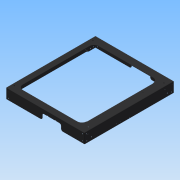
# Autodesk Inventor part: верхняя база
Saved by Autodesk Inventor 2017 (Build 210142000, 142)
## iProperties
Part Number: верхняя база
Material: Типовые
Document SubType Name: Modeling
Designer: Max
Mass: 130.784 g
Surface Area: 1912.46 cm^2
Volume: 130.784 cm^3
Density: 1 g/cm^3
Appearance: Резина — черная
Author: Max
Autodesk Inventor part; units mm, degrees
ref_plane "YZ Plane" through (0, 0, 0) normal (1, 0, 0) x (0, 1, 0)
ref_plane "XZ Plane" through (0, 0, 0) normal (0, 1, 0) x (-1, 0, 0)
ref_plane "XY Plane" through (0, 0, 0) normal (0, 0, 1) x (1, 0, 0)
sketch "Эскиз1" plane through (0, 0, 0) normal (0, 0, 1) x (1, 0, 0)
  line L0 (0, 0) -> (332.7, 0)
  line L1 (332.7, 0) -> (332.7, -378.7)
  line L2 (332.7, -378.7) -> (0, -378.7)
  line L3 (0, -378.7) -> (0, 0)
  line L4 (295.5, -31.2) -> (25, -31.2)
  line L5 (25, -31.2) -> (25, -352.7)
  line L6 (25, -352.7) -> (295.5, -352.7)
  line L7 (295.5, -352.7) -> (295.5, -31.2)
  line L8 (331.3, -1.4) -> (1.4, -1.4)
  line L9 (1.4, -1.4) -> (1.4, -377.3)
  line L10 (1.4, -377.3) -> (331.3, -377.3)
  line L11 (331.3, -377.3) -> (331.3, -1.4)
  dimension "d0" = 378.7
  dimension "d1" = 332.7
  dimension "d2" = 321.5
  dimension "d3" = 270.5
  dimension "d4" = 26
  dimension "d5" = 31.2
  dimension "d6" = 37.2
  dimension "d7" = 25
  dimension "d10" = 1.4
  constraints: 24 end point, 6 parallel, 3 perpendicular, 2 horizontal, 3 other
  measures "d0" distance between parallel lines of L2 L0
  measures "d1" distance between parallel lines of L3 L1
  measures "d2" distance between parallel lines of L4 L6
  measures "d3" distance between parallel lines of L5 L7
  measures "d4" distance between parallel lines of L2 L6
  measures "d5" distance between parallel lines of L0 L4
  measures "d6" distance between parallel lines of L7 L1
  measures "d7" distance between parallel lines of L3 L5
  measures "d10" distance between parallel lines of L0 L8
extrude "Выдавливание1" add sketch "Эскиз1" against normal blind 1.4 contours L0 L1 L2 L3 | L11 L10 L9 L8
extrude "Выдавливание2" add sketch "Эскиз1" against normal blind 42 contours L0 L1 L2 L3
fillet "Сопряжение1" radius 2 8 edges at (0, 0, -21) (166.35, 0, 0) (166.35, -378.7, 0) (0, -378.7, -21) (332.7, -378.7, -21) (332.7, -189.35, 0) (332.7, 0, -21) (0, -189.35, 0)
fillet "Сопряжение2" radius 0.6 8 edges at (1.4, -189.35, -1.4) (1.4, -1.4, -21.7) (166.35, -1.4, -1.4) (331.3, -1.4, -21.7) (331.3, -189.35, -1.4) (331.3, -377.3, -21.7) (1.4, -377.3, -21.7) (166.35, -377.3, -1.4)
sketch "Эскиз2" plane through (0, -376.7, -42) normal (-1, 0, 0) x (0, 0, 1)
  line L0 (0, 0) -> (0, 374.7) projected
  line L1 (0, 346.7) -> (4, 336.7)
  line L2 (4, 336.7) -> (4, 38)
  line L3 (4, 38) -> (0, 28)
  line L4 (0, 28) -> (0, 346.7)
  line L5 (40, 376.7) -> (0, 376.7) projected
  line L6 (0, -2) -> (40, -2) projected
  line L7 (42, 24) -> (42, 345.5) projected
  point P0 (42, 376.7)
  dimension "d15" = 30
  dimension "d16" = 40
  dimension "d17" = 30
  dimension "d18" = 40
  dimension "d19" = 38
  constraints: 8 end point, 2 parallel, 2 point on line
  measures "d15" distance from line of L1.start L5
  measures "d16" distance from line of L5 L1.end
  measures "d17" distance from line of L6 L3.end
  measures "d18" distance from line of L6 L2.end
  measures "d19" distance between parallel lines of L7 L2
extrude "Выдавливание3" cut sketch "Эскиз2" against normal blind 2
fillet "Сопряжение3" radius 10 4 edges at (0.7, -30, -42) (0.7, -40, -38) (0.7, -338.7, -38) (0.7, -348.7, -42)
sketch "Эскиз3" plane through (2, -378.7, -42) normal (0, -1, 0) x (1, 0, 0)
  line L0 (328.7, 0) -> (0, 0) projected
  line L1 (151.35, 0) -> (231.35, 0)
  line L2 (231.35, 0) -> (231.35, 24.5)
  line L3 (231.35, 24.5) -> (151.35, 24.5)
  line L4 (151.35, 24.5) -> (151.35, 0)
  line L5 (16.35, -307.35) -> (16.35, 42) projected
  line L6 (312.35, -307.35) -> (312.35, 42) projected
  circle A0 centre (174.35, 24.5) radius 2
  circle A1 centre (208.35, 24.5) radius 2
  point P0 (-2, 42)
  dimension "d23" = 135
  dimension "d24" = 81
  dimension "d25" = 24.5
  dimension "d26" = 80
  dimension "d30" = 4
  dimension "d31" = 4
  dimension "d32" = 34
  dimension "d33" = 23
  dimension "d34" = 23
  constraints: 8 end point, 3 point on line, 2 centre point, 2 parallel, 1 horizontal, 1 perpendicular
  measures "d23" distance between parallel lines of L5 L4
  measures "d24" distance between parallel lines of L6 L2
  measures "d25" distance between parallel lines of L0 L3
  measures "d26" distance between parallel lines of L2 L4
  measures "d30" diameter of A0
  measures "d31" diameter of A1
  measures "d32" distance of A1.centre A0.centre
  measures "d33" distance from line of L4 A0.centre
  measures "d34" distance of L2.end A1.centre
extrude "Выдавливание4" cut sketch "Эскиз3" against normal blind 500
fillet "Сопряжение4" radius 7 8 edges at (233.35, -378, -17.5) (233.35, -378, -42) (153.35, -378, -17.5) (153.35, -378, -42) (233.35, -0.7, -17.5) (233.35, -0.7, -42) (153.35, -0.7, -17.5) (153.35, -0.7, -42)
fillet "Сопряжение5" radius 20 4 edges at (25, -352.7, -0.7) (295.5, -352.7, -0.7) (295.5, -31.2, -0.7) (25, -31.2, -0.7)
sketch "Эскиз4" plane through (0, -376.7, -2) normal (-1, 0, 0) x (0, 0, 1)
  circle A0 centre (-6, 368.35) radius 2 projected
  circle A1 centre (-33, 366.35) radius 2 projected
  circle A2 centre (-6, 6.35) radius 2 projected
  circle A3 centre (-33, 8.35) radius 2 projected
  point P0 (2, 376.7)
extrude "Выдавливание5" cut sketch "Эскиз4" against normal blind 500
sketch "Эскиз5" plane through (2, -378.7, -2) normal (0, -1, 0) x (1, 0, 0)
  circle A0 centre (6.35, -6) radius 2 projected
  circle A1 centre (8.35, -33) radius 2 projected
  circle A2 centre (322.35, -6) radius 2 projected
  circle A3 centre (320.35, -33) radius 2 projected
  point P0 (-2, 2)
extrude "Выдавливание6" cut sketch "Эскиз5" against normal blind 500
sketch "Эскиз6" plane through (0, 0, -1.4) normal (0, 0, -1) x (-1, 0, 0)
  line L0 (-295.5, -332.7) -> (-295.5, -51.2) projected
  line L1 (-295.5, -51.2) -> (-296.9, -51.2)
  line L2 (-296.9, -51.2) -> (-296.9, -332.7)
  line L3 (-296.9, -332.7) -> (-295.5, -332.7)
  line L4 (-295.5, -332.7) -> (-295.5, -51.2)
  point P0 (0, 0)
  dimension "d40" = 1.4
  constraints: 8 end point, 2 parallel, 1 horizontal, 1 perpendicular
  measures "d40" distance between parallel lines of L0 L2
extrude "Выдавливание7" add sketch "Эскиз6" along normal blind 10.6
fillet "Сопряжение6" radius 4 2 edges at (296.2, -51.2, -12) (296.2, -332.7, -12)
sketch "Эскиз7" plane through (0, 0, 0) normal (0, 0, 1) x (1, 0, 0)
  line L0 (295.5, -55.2) -> (295.5, -51.2) projected
  line L1 (295.5, -51.2) -> (297.5, -51.2)
  line L2 (297.5, -51.2) -> (297.5, -51)
  line L3 (297.5, -51) -> (295.5, -51)
  line L4 (295.5, -51) -> (295.5, -51.2)
  line L5 (295.5, -51) -> (295.356, -51)
  line L6 (295.356, -51) -> (295.356, -51.2)
  line L7 (295.356, -51.2) -> (295.5, -51.2)
  line L8 (295.5, -51.2) -> (295.5, -51)
  line L9 (295.5, -332.7) -> (296.9, -332.7) projected
  line L10 (295.5, -332.7) -> (297.5, -332.7)
  line L11 (297.5, -332.7) -> (297.5, -332.9)
  line L12 (297.5, -332.9) -> (291.4104, -332.9)
  line L13 (291.4104, -332.9) -> (291.4104, -332.7)
  line L14 (291.4104, -332.7) -> (295.5, -332.7)
  line L15 (295.5, -51.2) -> (295.5, -332.7) projected
  point P0 (0, 0)
  dimension "d44" = 2
  dimension "d45" = 0.2
  dimension "d46" = 2
  dimension "d47" = 0.2
  constraints: 26 end point, 5 perpendicular, 4 parallel, 3 horizontal, 1 collinear
  measures "d44" distance of L3.end L2.end
  measures "d45" distance between parallel lines of L12 L9
  measures "d46" distance from line of L10.end L15
  measures "d47" distance between parallel lines of L1 L3
extrude "Выдавливание8" cut sketch "Эскиз7" against normal blind 10.6
fillet "Сопряжение7" radius 2 1 edges at (295.5, -191.95, 0)
sketch "Эскиз8" plane through (0, -376.7, -2) normal (-1, 0, 0) x (0, 0, 1)
  circle A0 centre (-10.5, 338.9) radius 1.5
  line L0 (2, 0) -> (2, 374.7) projected
  circle A1 centre (-10.5, 338.9) radius 4 construction
  line L1 (0, 376.7) -> (-40, 376.7) projected
  circle A2 centre (-10.5, 12.9) radius 1.5
  circle A3 centre (-10.5, 12.9) radius 4 construction
  point P0 (2, 376.7)
  dimension "d51" = 3
  dimension "d52" = 12.5
  dimension "d53" = 8
  dimension "d54" = 41.8
  dimension "d55" = 3
  dimension "d56" = 8
  dimension "d57" = 12.5
  dimension "d58" = 326
  dimension "d59" = 318
  constraints: 4 centre point, 2 coincident
  measures "d51" diameter of A0
  measures "d52" distance from line of A0.centre L0
  measures "d53" diameter of A1
  measures "d55" diameter of A2
  measures "d56" diameter of A3
  measures "d57" distance from line of L0 A2.centre
  measures "d58" distance of A0.centre A2.centre
extrude "Выдавливание9" cut sketch "Эскиз8" against normal blind 600
sketch "Эскиз9" plane through (0, -376.7, -2) normal (-1, 0, 0) x (0, 0, 1)
  line L0 (-11.5044, 298.2897) -> (-11.5044, -254.3895) construction
  line L1 (-11.5044, -254.3895) -> (-54.8278, -254.3895) construction
  line L2 (-54.8278, -254.3895) -> (-54.8278, 298.2897) construction
  line L3 (-54.8278, 298.2897) -> (-11.5044, 298.2897) construction
  line L4 (-11.7296, 296.9384) -> (-11.7296, 287.0164)
  line L5 (-11.7296, 287.0164) -> (-14.5198, 287.0164)
  line L6 (-14.5198, 287.0164) -> (-14.5198, 292.8971)
  line L7 (-14.5198, 292.8971) -> (-16.7844, 292.8971)
  line L8 (-16.7844, 292.8971) -> (-16.7844, 287.8797)
  line L9 (-16.7844, 287.8797) -> (-19.412, 287.8797)
  line L10 (-19.412, 287.8797) -> (-19.412, 292.8971)
  line L11 (-19.412, 292.8971) -> (-24.7296, 292.8971)
  line L12 (-24.7296, 292.8971) -> (-24.7296, 296.9384)
  line L13 (-24.7296, 296.9384) -> (-11.7296, 296.9384)
  line L14 (-11.7296, 284.8393) -> (-11.7296, 280.8229)
  line L15 (-11.7296, 280.8229) -> (-21.5265, 280.8229)
  line L16 (-21.5265, 280.8229) -> (-21.5265, 274.5544)
  line L17 (-21.5265, 274.5544) -> (-24.7296, 274.5544)
  line L18 (-24.7296, 274.5544) -> (-24.7296, 284.8393)
  line L19 (-24.7296, 284.8393) -> (-11.7296, 284.8393)
  line L20 (-11.7296, 274.0289) -> (-11.7296, 269.5621)
  line L21 (-11.7296, 269.5621) -> (-16.1088, 266.9471)
  line L22 (-16.1088, 266.9471) -> (-11.7296, 264.3196)
  line L23 (-11.7296, 264.3196) -> (-11.7296, 259.8778)
  line L24 (-11.7296, 259.8778) -> (-19.2869, 264.9327)
  line L25 (-19.2869, 264.9327) -> (-24.7296, 264.9327)
  line L26 (-24.7296, 264.9327) -> (-24.7296, 268.9615)
  line L27 (-24.7296, 268.9615) -> (-19.2869, 268.9615)
  line L28 (-19.2869, 268.9615) -> (-11.7296, 274.0289)
  line L29 (-11.7296, 258.4139) -> (-11.7296, 254.385)
  line L30 (-11.7296, 254.385) -> (-24.7296, 254.385)
  line L31 (-24.7296, 254.385) -> (-24.7296, 258.4139)
  line L32 (-24.7296, 258.4139) -> (-11.7296, 258.4139)
  line L33 (-11.7296, 251.4822) -> (-11.7296, 247.7286)
  line L34 (-11.7296, 247.7286) -> (-18.924, 242.8239)
  line L35 (-18.924, 242.8239) -> (-11.7296, 242.8239)
  line L36 (-11.7296, 242.8239) -> (-11.7296, 239.0328)
  line L37 (-11.7296, 239.0328) -> (-24.7296, 239.0328)
  line L38 (-24.7296, 239.0328) -> (-24.7296, 242.8239)
  line L39 (-24.7296, 242.8239) -> (-17.5727, 247.7036)
  line L40 (-17.5727, 247.7036) -> (-24.7296, 247.7036)
  line L41 (-24.7296, 247.7036) -> (-24.7296, 251.4822)
  line L42 (-24.7296, 251.4822) -> (-11.7296, 251.4822)
  line L43 (-20.0251, 229.8114) -> (-17.3225, 229.8114)
  line L44 (-17.3225, 229.8114) -> (-17.3225, 223.6054)
  line L45 (-17.3225, 223.6054) -> (-22.8528, 223.6054)
  spline S0 degree 2 poles (-22.8528, 223.6054) (-24.079, 225.3946) (-24.9548, 228.1348) (-24.9548, 230.0116) knots 0 0 0 1 2 2 2
  spline S1 degree 2 poles (-24.9548, 230.0116) (-24.9548, 232.3263) (-23.3783, 235.2541) (-20.2503, 236.8557) (-18.2233, 236.8557) knots 0 0 0 1 2 3 3 3
  spline S2 degree 2 poles (-18.2233, 236.8557) (-16.0963, 236.8557) (-12.9558, 235.104) (-12.13, 233.4023) knots 0 0 0 1 2 2 2
  spline S3 degree 2 poles (-12.13, 233.4023) (-11.5044, 232.0761) (-11.5044, 229.8489) knots 0 0 0 1 1 1
  spline S4 degree 2 poles (-11.5044, 229.8489) (-11.5044, 227.6844) (-12.2801, 225.5448) (-13.9317, 224.1309) (-15.1829, 223.7806) knots 0 0 0 1 2 3 3 3
  line L46 (-15.1829, 223.7806) -> (-15.8836, 227.6593)
  spline S5 degree 2 poles (-15.8836, 227.6593) (-15.1454, 227.8971) (-14.3571, 229.0482) (-14.3571, 229.9365) knots 0 0 0 1 2 2 2
  spline S6 degree 2 poles (-14.3571, 229.9365) (-14.3571, 231.2503) (-16.1964, 232.8268) (-18.1858, 232.8268) knots 0 0 0 1 2 2 2
  spline S7 degree 2 poles (-18.1858, 232.8268) (-20.2878, 232.8268) (-22.1021, 231.2378) (-22.1021, 229.8114) knots 0 0 0 1 2 2 2
  spline S8 degree 2 poles (-22.1021, 229.8114) (-22.1021, 229.1357) (-21.7142, 227.9096) (-21.2387, 227.1213) knots 0 0 0 1 2 2 2
  line L47 (-21.2387, 227.1213) -> (-20.0251, 227.1213)
  line L48 (-20.0251, 227.1213) -> (-20.0251, 229.8114)
  line L49 (-11.7296, 215.1598) -> (-11.7296, 207.6401)
  spline S9 degree 2 poles (-11.7296, 207.6401) (-11.7296, 205.7633) (-13.5939, 203.7488) (-14.9702, 203.7488) knots 0 0 0 1 2 2 2
  spline S10 degree 2 poles (-14.9702, 203.7488) (-16.1213, 203.7488) (-16.9471, 204.462) knots 0 0 0 1 1 1
  spline S11 degree 2 poles (-16.9471, 204.462) (-17.4976, 204.95) (-17.8229, 205.8759) knots 0 0 0 1 1 1
  spline S12 degree 2 poles (-17.8229, 205.8759) (-18.1608, 204.4745) (-19.7998, 203.1483) (-21.0385, 203.1483) knots 0 0 0 1 2 2 2
  spline S13 degree 2 poles (-21.0385, 203.1483) (-22.0395, 203.1483) (-23.6536, 204.0867) (-24.129, 204.8999) knots 0 0 0 1 2 2 2
  spline S14 degree 2 poles (-24.129, 204.8999) (-24.4168, 205.4129) (-24.5544, 206.4264) knots 0 0 0 1 1 1
  spline S15 degree 2 poles (-24.5544, 206.4264) (-24.7296, 207.7902) (-24.7296, 208.2281) knots 0 0 0 1 1 1
  line L50 (-24.7296, 208.2281) -> (-24.7296, 215.1598)
  line L51 (-24.7296, 215.1598) -> (-11.7296, 215.1598)
  line L52 (-21.9394, 211.1059) -> (-21.9394, 209.0664)
  spline S16 degree 2 poles (-21.9394, 209.0664) (-21.9394, 208.028) (-21.2012, 207.1771) (-20.5881, 207.1771) knots 0 0 0 1 2 2 2
  spline S17 degree 2 poles (-20.5881, 207.1771) (-20.0126, 207.1771) (-19.3119, 208.0154) (-19.3119, 209.0664) knots 0 0 0 1 2 2 2
  line L53 (-19.3119, 209.0664) -> (-19.3119, 211.1059)
  line L54 (-19.3119, 211.1059) -> (-21.9394, 211.1059)
  line L55 (-16.8345, 211.1059) -> (-16.8345, 209.3667)
  spline S18 degree 2 poles (-16.8345, 209.3667) (-16.8345, 208.4283) (-16.1839, 207.6901) (-15.5708, 207.6901) knots 0 0 0 1 2 2 2
  spline S19 degree 2 poles (-15.5708, 207.6901) (-15.0077, 207.6901) (-14.3696, 208.4283) (-14.3696, 209.3417) knots 0 0 0 1 2 2 2
  line L56 (-14.3696, 209.3417) -> (-14.3696, 211.1059)
  line L57 (-14.3696, 211.1059) -> (-16.8345, 211.1059)
  line L58 (-11.7296, 201.0337) -> (-11.7296, 190.2734)
  line L59 (-11.7296, 190.2734) -> (-14.5073, 190.2734)
  line L60 (-14.5073, 190.2734) -> (-14.5073, 197.0049)
  line L61 (-14.5073, 197.0049) -> (-16.5717, 197.0049)
  line L62 (-16.5717, 197.0049) -> (-16.5717, 190.7613)
  line L63 (-16.5717, 190.7613) -> (-19.2243, 190.7613)
  line L64 (-19.2243, 190.7613) -> (-19.2243, 197.0049)
  line L65 (-19.2243, 197.0049) -> (-21.7893, 197.0049)
  line L66 (-21.7893, 197.0049) -> (-21.7893, 190.0732)
  line L67 (-21.7893, 190.0732) -> (-24.7296, 190.0732)
  line L68 (-24.7296, 190.0732) -> (-24.7296, 201.0337)
  line L69 (-24.7296, 201.0337) -> (-11.7296, 201.0337)
  line L70 (-22.5775, 179.9134) -> (-22.5775, 184.4803)
  line L71 (-22.5775, 184.4803) -> (-24.7296, 185.1184)
  line L72 (-24.7296, 185.1184) -> (-24.7296, 189.2224)
  line L73 (-24.7296, 189.2224) -> (-11.7296, 184.3302)
  line L74 (-11.7296, 184.3302) -> (-11.7296, 179.9384)
  line L75 (-11.7296, 179.9384) -> (-24.7296, 175.0588)
  line L76 (-24.7296, 175.0588) -> (-24.7296, 179.2628)
  line L77 (-24.7296, 179.2628) -> (-22.5775, 179.9134)
  line L78 (-19.7623, 180.7517) -> (-15.0953, 182.1781)
  line L79 (-15.0953, 182.1781) -> (-19.7623, 183.6045)
  line L80 (-19.7623, 183.6045) -> (-19.7623, 180.7517)
  line L81 (-24.7296, 173.7075) -> (-11.7296, 173.7075)
  line L82 (-11.7296, 173.7075) -> (-11.7296, 167.0135)
  spline S20 degree 2 poles (-11.7296, 167.0135) (-11.7296, 165.1617) (-12.3677, 163.1848) (-14.0944, 161.9837) (-15.3331, 161.9837) knots 0 0 0 1 2 3 3 3
  spline S21 degree 2 poles (-15.3331, 161.9837) (-16.4216, 161.9837) (-17.9856, 162.9096) (-18.4736, 163.7103) knots 0 0 0 1 2 2 2
  spline S22 degree 2 poles (-18.4736, 163.7103) (-18.7864, 164.2233) (-18.9866, 165.1242) knots 0 0 0 1 1 1
  spline S23 degree 2 poles (-18.9866, 165.1242) (-19.2243, 164.411) (-19.462, 164.0732) knots 0 0 0 1 1 1
  spline S24 degree 2 poles (-19.462, 164.0732) (-19.6247, 163.8605) (-20.6757, 163.0222) (-20.9635, 162.872) knots 0 0 0 1 2 2 2
  line L83 (-20.9635, 162.872) -> (-24.7296, 160.9327)
  line L84 (-24.7296, 160.9327) -> (-24.7296, 165.4745)
  line L85 (-24.7296, 165.4745) -> (-20.7508, 167.6141)
  spline S25 degree 2 poles (-20.7508, 167.6141) (-19.9875, 168.0145) (-19.7498, 168.3273) knots 0 0 0 1 1 1
  spline S26 degree 2 poles (-19.7498, 168.3273) (-19.4495, 168.7652) (-19.4495, 169.3157) knots 0 0 0 1 1 1
  line L86 (-19.4495, 169.3157) -> (-19.4495, 169.6661)
  line L87 (-19.4495, 169.6661) -> (-24.7296, 169.6661)
  line L88 (-24.7296, 169.6661) -> (-24.7296, 173.7075)
  line L89 (-16.9972, 169.6661) -> (-16.9972, 167.9769)
  spline S27 degree 2 poles (-16.9972, 167.9769) (-16.9972, 167.7142) (-16.822, 166.9259) knots 0 0 0 1 1 1
  spline S28 degree 2 poles (-16.822, 166.9259) (-16.7344, 166.5255) (-16.0838, 166.0251) (-15.6584, 166.0251) knots 0 0 0 1 2 2 2
  spline S29 degree 2 poles (-15.6584, 166.0251) (-15.0328, 166.0251) (-14.3571, 166.8133) (-14.3571, 167.9144) knots 0 0 0 1 2 2 2
  line L90 (-14.3571, 167.9144) -> (-14.3571, 169.6661)
  line L91 (-14.3571, 169.6661) -> (-16.9972, 169.6661)
  line L92 (-20.0251, 147.0193) -> (-17.3225, 147.0193)
  line L93 (-17.3225, 147.0193) -> (-17.3225, 140.8133)
  line L94 (-17.3225, 140.8133) -> (-22.8528, 140.8133)
  spline S30 degree 2 poles (-22.8528, 140.8133) (-24.079, 142.6025) (-24.9548, 145.3427) (-24.9548, 147.2195) knots 0 0 0 1 2 2 2
  spline S31 degree 2 poles (-24.9548, 147.2195) (-24.9548, 149.5342) (-23.3783, 152.462) (-20.2503, 154.0636) (-18.2233, 154.0636) knots 0 0 0 1 2 3 3 3
  spline S32 degree 2 poles (-18.2233, 154.0636) (-16.0963, 154.0636) (-12.9558, 152.3119) (-12.13, 150.6102) knots 0 0 0 1 2 2 2
  spline S33 degree 2 poles (-12.13, 150.6102) (-11.5044, 149.284) (-11.5044, 147.0568) knots 0 0 0 1 1 1
  spline S34 degree 2 poles (-11.5044, 147.0568) (-11.5044, 144.8922) (-12.2801, 142.7527) (-13.9317, 141.3388) (-15.1829, 140.9885) knots 0 0 0 1 2 3 3 3
  line L95 (-15.1829, 140.9885) -> (-15.8836, 144.8672)
  spline S35 degree 2 poles (-15.8836, 144.8672) (-15.1454, 145.105) (-14.3571, 146.2561) (-14.3571, 147.1444) knots 0 0 0 1 2 2 2
  spline S36 degree 2 poles (-14.3571, 147.1444) (-14.3571, 148.4582) (-16.1964, 150.0347) (-18.1858, 150.0347) knots 0 0 0 1 2 2 2
  spline S37 degree 2 poles (-18.1858, 150.0347) (-20.2878, 150.0347) (-22.1021, 148.4457) (-22.1021, 147.0193) knots 0 0 0 1 2 2 2
  spline S38 degree 2 poles (-22.1021, 147.0193) (-22.1021, 146.3436) (-21.7142, 145.1175) (-21.2387, 144.3292) knots 0 0 0 1 2 2 2
  line L96 (-21.2387, 144.3292) -> (-20.0251, 144.3292)
  line L97 (-20.0251, 144.3292) -> (-20.0251, 147.0193)
  line L98 (-11.7296, 138.411) -> (-11.7296, 134.3947)
  line L99 (-11.7296, 134.3947) -> (-16.284, 134.3947)
  line L100 (-16.284, 134.3947) -> (-16.284, 130.0029)
  line L101 (-16.284, 130.0029) -> (-11.7296, 130.0029)
  line L102 (-11.7296, 130.0029) -> (-11.7296, 125.9615)
  line L103 (-11.7296, 125.9615) -> (-24.7296, 125.9615)
  line L104 (-24.7296, 125.9615) -> (-24.7296, 130.0029)
  line L105 (-24.7296, 130.0029) -> (-19.4745, 130.0029)
  line L106 (-19.4745, 130.0029) -> (-19.4745, 134.3947)
  line L107 (-19.4745, 134.3947) -> (-24.7296, 134.3947)
  line L108 (-24.7296, 134.3947) -> (-24.7296, 138.411)
  line L109 (-24.7296, 138.411) -> (-11.7296, 138.411)
  spline S39 degree 2 poles (-18.2358, 123.797) (-15.0578, 123.797) (-11.5044, 120.2435) (-11.5044, 117.078) knots 0 0 0 1 2 2 2
  spline S40 degree 2 poles (-11.5044, 117.078) (-11.5044, 113.8374) (-14.9952, 110.3215) (-18.1357, 110.3215) knots 0 0 0 1 2 2 2
  spline S41 degree 2 poles (-18.1357, 110.3215) (-20.4129, 110.3215) (-23.3282, 111.8605) (-24.9548, 114.7633) (-24.9548, 116.9279) knots 0 0 0 1 2 3 3 3
  spline S42 degree 2 poles (-24.9548, 116.9279) (-24.9548, 119.1175) (-23.5535, 122.0077) (-20.513, 123.797) (-18.2358, 123.797) knots 0 0 0 1 2 3 3 3
  spline S43 degree 2 poles (-18.2609, 119.7806) (-20.2253, 119.7806) (-21.9519, 118.3167) (-21.9519, 117.053) knots 0 0 0 1 2 2 2
  spline S44 degree 2 poles (-21.9519, 117.053) (-21.9519, 115.7642) (-20.2628, 114.3379) (-18.0857, 114.3379) knots 0 0 0 1 2 2 2
  spline S45 degree 2 poles (-18.0857, 114.3379) (-16.2464, 114.3379) (-14.5448, 115.8143) (-14.5448, 117.0905) knots 0 0 0 1 2 2 2
  spline S46 degree 2 poles (-14.5448, 117.0905) (-14.5448, 118.3042) (-16.2715, 119.7806) (-18.2609, 119.7806) knots 0 0 0 1 2 2 2
  line L110 (-20.4254, 108.8576) -> (-20.1877, 105.0289)
  spline S47 degree 2 poles (-20.1877, 105.0289) (-21.1261, 104.9038) (-21.6141, 104.5284) knots 0 0 0 1 1 1
  spline S48 degree 2 poles (-21.6141, 104.5284) (-22.4023, 103.9028) (-22.4023, 102.7392) knots 0 0 0 1 1 1
  spline S49 degree 2 poles (-22.4023, 102.7392) (-22.4023, 101.8884) (-21.5891, 100.95) (-21.0636, 100.95) knots 0 0 0 1 2 2 2
  spline S50 degree 2 poles (-21.0636, 100.95) (-20.5631, 100.95) (-20.1627, 101.4004) knots 0 0 0 1 1 1
  spline S51 degree 2 poles (-20.1627, 101.4004) (-19.7623, 101.8383) (-19.3995, 103.4524) knots 0 0 0 1 1 1
  spline S52 degree 2 poles (-19.3995, 103.4524) (-18.8114, 106.105) (-17.8229, 107.231) knots 0 0 0 1 1 1
  spline S53 degree 2 poles (-17.8229, 107.231) (-16.8345, 108.3696) (-15.308, 108.3696) knots 0 0 0 1 1 1
  spline S54 degree 2 poles (-15.308, 108.3696) (-14.3071, 108.3696) (-12.5304, 107.206) (-11.5044, 104.8663) (-11.5044, 102.8393) knots 0 0 0 1 2 3 3 3
  spline S55 degree 2 poles (-11.5044, 102.8393) (-11.5044, 100.3369) (-13.3562, 97.7219) (-15.3831, 97.4717) knots 0 0 0 1 2 2 2
  line L111 (-15.3831, 97.4717) -> (-15.6083, 101.2628)
  spline S56 degree 2 poles (-15.6083, 101.2628) (-14.7325, 101.4129) (-13.9317, 102.3889) (-13.9317, 103.2397) knots 0 0 0 1 2 2 2
  spline S57 degree 2 poles (-13.9317, 103.2397) (-13.9317, 103.9404) (-14.5198, 104.6536) (-14.9577, 104.6536) knots 0 0 0 1 2 2 2
  spline S58 degree 2 poles (-14.9577, 104.6536) (-15.258, 104.6536) (-15.5082, 104.3533) knots 0 0 0 1 1 1
  spline S59 degree 2 poles (-15.5082, 104.3533) (-15.771, 104.0655) (-15.9837, 103.002) knots 0 0 0 1 1 1
  spline S60 degree 2 poles (-15.9837, 103.002) (-16.5592, 100.3619) (-17.7229, 98.0847) (-19.437, 97.0462) (-20.5005, 97.0462) knots 0 0 0 1 2 3 3 3
  spline S61 degree 2 poles (-20.5005, 97.0462) (-21.7517, 97.0462) (-23.8663, 98.4351) (-24.9548, 100.9125) (-24.9548, 102.8143) knots 0 0 0 1 2 3 3 3
  spline S62 degree 2 poles (-24.9548, 102.8143) (-24.9548, 106.13) (-22.4023, 108.6949) (-20.4254, 108.8576) knots 0 0 0 1 2 2 2
  line L112 (-11.7296, 95.9452) -> (-11.7296, 83.7209)
  line L113 (-11.7296, 83.7209) -> (-14.9452, 83.7209)
  line L114 (-14.9452, 83.7209) -> (-14.9452, 87.8249)
  line L115 (-14.9452, 87.8249) -> (-24.7296, 87.8249)
  line L116 (-24.7296, 87.8249) -> (-24.7296, 91.8412)
  line L117 (-24.7296, 91.8412) -> (-14.9452, 91.8412)
  line L118 (-14.9452, 91.8412) -> (-14.9452, 95.9452)
  line L119 (-14.9452, 95.9452) -> (-11.7296, 95.9452)
  line L120 (-11.7296, 74.9625) -> (-11.7296, 66.4043)
  line L121 (-11.7296, 66.4043) -> (-14.6074, 66.4043)
  line L122 (-14.6074, 66.4043) -> (-14.6074, 72.1973)
  line L123 (-14.6074, 72.1973) -> (-16.5592, 72.4976)
  spline S63 degree 2 poles (-16.5592, 72.4976) (-16.284, 71.8971) (-15.9962, 70.7209) (-15.9962, 70.1454) knots 0 0 0 1 2 2 2
  spline S64 degree 2 poles (-15.9962, 70.1454) (-15.9962, 68.206) (-18.361, 65.7787) (-20.1502, 65.7787) knots 0 0 0 1 2 2 2
  spline S65 degree 2 poles (-20.1502, 65.7787) (-21.4014, 65.7787) (-23.7286, 67.0299) (-24.9548, 69.3196) (-24.9548, 71.1088) knots 0 0 0 1 2 3 3 3
  spline S66 degree 2 poles (-24.9548, 71.1088) (-24.9548, 72.3975) (-24.4668, 74.2243) (-23.5034, 75.513) (-22.2772, 76.3138) (-21.3639, 76.5766) knots 0 0 0 1 2 3 4 4 4
  line L124 (-21.3639, 76.5766) -> (-20.9635, 72.923)
  spline S67 degree 2 poles (-20.9635, 72.923) (-21.8393, 72.7854) (-22.7527, 71.822) (-22.7527, 71.1463) knots 0 0 0 1 2 2 2
  spline S68 degree 2 poles (-22.7527, 71.1463) (-22.7527, 70.3956) (-21.6141, 69.4197) (-20.4755, 69.4197) knots 0 0 0 1 2 2 2
  spline S69 degree 2 poles (-20.4755, 69.4197) (-19.3119, 69.4197) (-18.2358, 70.4081) (-18.2358, 71.2214) knots 0 0 0 1 2 2 2
  spline S70 degree 2 poles (-18.2358, 71.2214) (-18.2358, 71.7469) (-18.4986, 72.2349) knots 0 0 0 1 1 1
  spline S71 degree 2 poles (-18.4986, 72.2349) (-18.6738, 72.5852) (-19.1617, 73.0231) knots 0 0 0 1 1 1
  line L125 (-19.1617, 73.0231) -> (-18.7238, 76.1011)
  line L126 (-18.7238, 76.1011) -> (-11.7296, 74.9625)
  point P0 (2, 376.7)
  constraints: 2 other
extrude "Выдавливание10" add sketch "Эскиз9" along normal blind 0.1
sketch "Эскиз10" plane through (0, 0, 0) normal (0, 0, 1) x (1, 0, 0)
  circle A0 centre (308.35, -96.85) radius 6 projected
  circle A1 centre (308.35, -107.85) radius 1.5 projected
  circle A2 centre (308.35, -85.85) radius 1.5 projected
  circle A3 centre (308.35, -270.85) radius 1.5 projected
  circle A4 centre (308.35, -281.85) radius 6 projected
  circle A5 centre (308.35, -292.85) radius 1.5 projected
  line L0 (315.25, -295.85) -> (301.45, -295.85) projected
  line L1 (315.25, -110.85) -> (301.45, -110.85) projected
  line L2 (300.95, -110.35) -> (300.95, -83.35) projected
  line L3 (300.95, -295.35) -> (300.95, -268.35) projected
  line L4 (315.75, -268.35) -> (315.75, -295.35) projected
  line L5 (301.45, -267.85) -> (315.25, -267.85) projected
  line L6 (315.75, -83.35) -> (315.75, -110.35) projected
  line L7 (301.45, -82.85) -> (315.25, -82.85) projected
  point P0 (0, 0)
extrude "Выдавливание11" cut sketch "Эскиз10" against normal blind 5 contours A1 | A2 | A3 | A5
sketch "Эскиз11" plane through (0, -376.7, -2) normal (-1, 0, 0) x (0, 0, 1)
  circle A0 centre (-33.5, 354.7) radius 2
  circle A1 centre (-33.5, 21.7) radius 2
  line L0 (0, 376.7) -> (-40, 376.7) projected
  line L1 (-40, -2) -> (0, -2) projected
  line L2 (-47.7633, 16.35) -> (-56.1519, 16.35)
  line L3 (2, 0) -> (2, 374.7) projected
  point P0 (2, 376.7)
  dimension "d66" = 4
  dimension "d67" = 4
  dimension "d68" = 22
  dimension "d70" = 333
  dimension "d71" = 5.35
  dimension "d73" = 18.35
  dimension "d74" = 35.5
  dimension "d75" = 35.5
  dimension "d78" = 23.7
  constraints: 2 centre point, 2 end point, 1 horizontal
  measures "d66" diameter of A0
  measures "d67" diameter of A1
  measures "d68" distance from line of L0 A0.centre
  measures "d70" distance of A0.centre A1.centre
  measures "d71" distance from line of L2 A1.centre
  measures "d73" distance between parallel lines of L1 L2
  measures "d74" distance from line of A0.centre L3
  measures "d75" distance from line of L3 A1.centre
  measures "d78" distance from line of A1.centre L1
extrude "Выдавливание12" cut sketch "Эскиз11" against normal blind 5
sketch "Эскиз12" plane through (0, 0, 0) normal (0, 0, 1) x (1, 0, 0)
  circle A0 centre (11.5, -22) radius 2
  circle A1 centre (11.5, -355) radius 2
  line L0 (330.7, 0) -> (2, 0) projected
  line L1 (2, -378.7) -> (330.7, -378.7) projected
  line L2 (0, -2) -> (0, -376.7) projected
  circle A2 centre (318.2, -28) radius 2
  circle A3 centre (318.2, -348.7) radius 2
  line L3 (332.7, -376.7) -> (332.7, -2) projected
  point P0 (0, 0)
  dimension "d79" = 4
  dimension "d80" = 4
  dimension "d81" = 22
  dimension "d82" = 23.7
  dimension "d83" = 333
  dimension "d84" = 11.5
  dimension "d85" = 11.5
  dimension "d86" = 4
  dimension "d87" = 4
  dimension "d88" = 14.5
  dimension "d89" = 14.5
  dimension "d90" = 28
  dimension "d91" = 30
  constraints: 4 centre point
  measures "d79" diameter of A0
  measures "d80" diameter of A1
  measures "d81" distance from line of L0 A0.centre
  measures "d82" distance from line of L1 A1.centre
  measures "d83" distance of A0.centre A1.centre
  measures "d84" distance from line of L2 A0.centre
  measures "d85" distance from line of L2 A1.centre
  measures "d86" diameter of A2
  measures "d87" diameter of A3
  measures "d88" distance from line of L3 A3.centre
  measures "d89" distance from line of L3 A2.centre
  measures "d90" distance from line of L0 A2.centre
  measures "d91" distance from line of L1 A3.centre
extrude "Выдавливание13" cut sketch "Эскиз12" against normal blind 5
sketch "Эскиз13" plane through (332.7, -376.7, -2) normal (1, 0, 0) x (0, 0, -1)
  circle A0 centre (28, 348.7) radius 2
  line L0 (40, 376.7) -> (0, 376.7) projected
  line L1 (-2, 374.7) -> (-2, 0) projected
  circle A1 centre (28, 28) radius 2
  line L2 (0, -2) -> (40, -2) projected
  point P0 (-2, 376.7)
  dimension "d94" = 4
  dimension "d95" = 28
  dimension "d96" = 30
  dimension "d97" = 4
  dimension "d98" = 30
  dimension "d99" = 30
  constraints: 2 centre point
  measures "d94" diameter of A0
  measures "d95" distance from line of L0 A0.centre
  measures "d96" distance from line of L1 A0.centre
  measures "d97" diameter of A1
  measures "d98" distance from line of L2 A1.centre
  measures "d99" distance from line of A1.centre L1
extrude "Выдавливание14" cut sketch "Эскиз13" against normal blind 5
sketch "Эскиз14" plane through (1.4, -376.7, -2) normal (1, 0, 0) x (0, 0, -1)
  circle A0 centre (25.0596, 330.9914) radius 1.5 projected
  circle A1 centre (25.0596, 330.9914) radius 1
  point P0 (-2, 376.7)
  dimension "d104" = 2
  constraints: 1 centre point, 1 coincident
  measures "d104" diameter of A1
extrude "Выдавливание15" add sketch "Эскиз14" along normal blind 12
sketch "Эскиз15" plane through (332.7, -376.7, -2) normal (1, 0, 0) x (0, 0, -1)
  circle A0 centre (34, 135) radius 1.5
  circle A1 centre (34, 150) radius 1.5
  line L0 (-2, 374.7) -> (-2, 0) projected
  line L1 (0, -2) -> (40, -2) projected
  point P0 (-2, 376.7)
  dimension "d105" = 3
  dimension "d106" = 3
  dimension "d107" = 36
  dimension "d108" = 36
  dimension "d109" = 15
  dimension "d110" = 137
  constraints: 2 centre point
  measures "d105" diameter of A0
  measures "d106" diameter of A1
  measures "d107" distance from line of A1.centre L0
  measures "d108" distance from line of L0 A0.centre
  measures "d109" distance of A1.centre A0.centre
  measures "d110" distance from line of L1 A0.centre
extrude "Выдавливание16" cut sketch "Эскиз15" against normal blind 12
sketch "Эскиз16" plane through (332.7, -376.7, -2) normal (1, 0, 0) x (0, 0, -1)
  circle A0 centre (37, 187.85) radius 1.5
  line L0 (-2, 374.7) -> (-2, 0) projected
  circle A1 centre (45, 366.85) radius 1.1293 projected
  circle A2 centre (10.5, 338.9) radius 1.5 projected
  circle A3 centre (34, 150) radius 1.5 projected
  point P0 (-2, 376.7)
  dimension "d113" = 3
  dimension "d114" = 39
  dimension "d115" = 179
  dimension "d116" = 151.05
  dimension "d119" = 36
  constraints: 1 centre point
  measures "d113" diameter of A0
  measures "d114" distance from line of L0 A0.centre
  measures "d115" vertical distance of A0.centre A1.centre
  measures "d116" vertical distance of A0.centre A2.centre
  measures "d119" distance from line of L0 A3.centre
extrude "Выдавливание17" cut sketch "Эскиз16" against normal blind 10 contours A0
